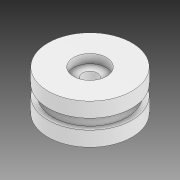
# Autodesk Inventor part: 1213_Distal Roller_V1
Saved by Autodesk Inventor 2020 (Build 240168000, 168)
## iProperties
Created: 2019-09-26
Part Number: 1213_Distal Roller_V1
Material: Acetal Resin, White
Document SubType Name: Modeling
Designer: MPI
Density: 1.425 g/cm^3
Appearance: Smooth - White
Author: MPI
Autodesk Inventor part; units mm, degrees
ref_plane "YZ Plane" through (0, 0, 0) normal (1, 0, 0) x (0, 1, 0)
ref_plane "XZ Plane" through (0, 0, 0) normal (0, 1, 0) x (-1, 0, 0)
ref_plane "XY Plane" through (0, 0, 0) normal (0, 0, 1) x (1, 0, 0)
sketch "Sketch1" plane through (0, 0, 0) normal (0, 0, 1) x (1, 0, 0)
  line L0 (0, 0) -> (0, 20.9396) construction
  line L1 (5, 0) -> (28.3, 0)
  line L2 (28.3, 0) -> (28.3, 10)
  line L3 (28.3, 10) -> (25, 10)
  line L4 (25, 10) -> (25, 17)
  line L5 (25, 17) -> (28.3, 17)
  line L6 (28.3, 17) -> (28.3, 27)
  line L7 (28.3, 27) -> (5, 27)
  line L8 (5, 27) -> (5, 0)
  dimension "d1" = 3.3
  dimension "d2" = 7
  dimension "d4" = 10
  dimension "d15" = 25
  dimension "d16" = 5
  constraints: 18 end point, 5 perpendicular, 3 point on line, 2 vertical, 1 collinear
  measures "d1" distance of L4.end L5.end
  measures "d2" distance of L3.end L4.end
  measures "d4" distance of L5.end L6.end
  measures "d15" distance between parallel lines of L0 L4
  measures "d16" distance between parallel lines of L8 L0
revolve "Revolution1" add sketch "Sketch1" angle 360 about axis through (0, 0, 0) along (0, 1, 0)
sketch "Sketch2" plane through (0, 27, 0) normal (0, 1, 0) x (1, 0, 0)
  circle A0 centre (0, 0) radius 11.15
  dimension "d8" = 22.3
  constraints: 1 centre point, 1 coincident
  measures "d8" diameter of A0
extrude "Extrusion1" cut sketch "Sketch2" against normal blind 6
sketch "Sketch3" plane through (0, 0, 0) normal (0, -1, 0) x (1, 0, 0)
  circle A0 centre (0, 0) radius 11.15
  dimension "d11" = 22.3
  constraints: 1 centre point, 1 coincident
  measures "d11" diameter of A0
extrude "Extrusion2" cut sketch "Sketch3" against normal blind 6
body "Solid1"
